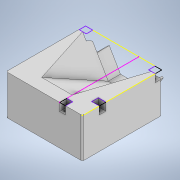
# Autodesk Inventor part: pipet tip trough
Saved by Autodesk Inventor 2020 (Build 240168000, 168)
## iProperties
Created: 2021-10-10
Part Number: pipet tip trough
Material: Generic
Document SubType Name: Modeling
Designer: pab2
Density: 1 g/cm^3
Appearance: Default
Author: pab2
Autodesk Inventor part; units mm, degrees
ref_plane "YZ Plane" through (0, 0, 0) normal (1, 0, 0) x (0, 1, 0)
ref_plane "XZ Plane" through (0, 0, 0) normal (0, 1, 0) x (-1, 0, 0)
ref_plane "XY Plane" through (0, 0, 0) normal (0, 0, 1) x (1, 0, 0)
sketch "Sketch1" plane through (0, 0, 0) normal (0, 1, 0) x (-1, 0, 0)
  line L0 (3.175, 0) -> (155.575, 0)
  line L1 (158.75, -3.175) -> (158.75, -161.925)
  line L2 (155.575, -165.1) -> (3.175, -165.1)
  line L3 (0, -161.925) -> (0, -3.175)
  arc A0 (158.75, -3.175) -> (155.575, 0) centre (155.575, -3.175) ccw
  arc A1 (155.575, -165.1) -> (158.75, -161.925) centre (155.575, -161.925) ccw
  arc A2 (0, -161.925) -> (3.175, -165.1) centre (3.175, -161.925) ccw
  arc A3 (3.175, 0) -> (0, -3.175) centre (3.175, -3.175) ccw
  point P0 (0, 0)
  point P1 (158.75, -165.1)
  point P2 (158.75, 0)
  point P3 (0, -165.1)
  dimension "d0" = 158.75
  dimension "d1" = 165.1
  dimension "d2" = 3.175
  dimension "d3" = 3.175
  dimension "d4" = 3.175
  dimension "d5" = 3.175
  constraints: 8 end point, 8 point on circle, 8 point on line, 8 tangent, 4 centre point, 2 parallel, 1 horizontal, 1 perpendicular
  measures "d0" distance of point (158.75, -165.1) point (0, -165.1)
  measures "d1" distance of point (158.75, 0) point (158.75, -165.1)
  measures "d2" radius of A0
  measures "d3" radius of A1
  measures "d4" radius of A2
  measures "d5" radius of A3
extrude "Extrusion1" add sketch "Sketch1" along normal blind 82.55
sketch "Sketch2" plane through (0, 0, 0) normal (0, -1, 0) x (1, 0, 0)
  line L0 (-3.175, -165.1) -> (-155.575, -165.1) projected
  line L1 (-6.5142, -165.1) -> (0, -165.1)
  line L2 (0, -158.9917) -> (0, -165.1)
  line L3 (0, -165.1) -> (-7.9375, -165.1)
  line L4 (-7.9375, -165.1) -> (-7.9375, -157.1625)
  line L5 (-7.9375, -157.1625) -> (0, -157.1625)
  line L6 (0, -157.1625) -> (0, -165.1)
  line L7 (-7.9375, -157.1625) -> (-149.225, -157.1625)
  line L8 (-7.9375, -157.1625) -> (-7.9375, -41.275)
  line L9 (-7.9375, -41.275) -> (-42.5857, -6.6268)
  line L10 (-7.9375, -41.275) -> (41.0625, -41.275) construction
  point P0 (0, 0)
  dimension "d8" = 7.9375
  dimension "d9" = 7.9375
  dimension "d10" = 141.2875
  dimension "d11" = 115.8875
  dimension "d12" = 49
  dimension "d13" = 135
  constraints: 20 end point, 3 horizontal, 2 parallel, 2 vertical, 1 collinear, 1 equal length, 1 perpendicular, 1 point on line
  measures "d8" distance of L4.end L5.end
  measures "d9" distance of L3.end L4.end
  measures "d10" distance of L4.end L7.end
  measures "d11" distance of L4.end L8.end
  measures "d12" distance of L8.end L9.end
  measures "d13" angle of L10 L9
hole "Hole1" at (-42.5857, 0, -6.6268) at (-7.9375, 0, -41.275) at (-7.9375, 0, -157.1625) at (-149.225, 0, -157.1625) direction (0, 1, 0) diameter 4.7625 end through all
sketch "Sketch7" plane through (-3.175, 0, -165.1) normal (0, 0, -1) x (-1, 0, 0)
  line L0 (0, 0) -> (0, 82.55) projected
  line L1 (0, 82.55) -> (44.45, 82.55)
  line L2 (152.4, 82.55) -> (0, 82.55) projected
  line L3 (0, 82.55) -> (44.45, 82.55) construction
  line L4 (44.45, 82.55) -> (107.95, 82.55)
  line L5 (107.95, 82.55) -> (107.95, 6.35)
  line L6 (107.95, 6.35) -> (44.45, 6.35)
  line L7 (44.45, 6.35) -> (44.45, 82.55)
  line L8 (44.45, 6.35) -> (0, 82.55)
  line L9 (107.95, 6.35) -> (152.4, 82.55)
  line L10 (107.95, 82.55) -> (152.4, 82.55)
  point P0 (-3.175, 0)
  dimension "d22" = 44.45
  dimension "d23" = 0
  dimension "d24" = 63.5
  dimension "d25" = 76.2
  constraints: 18 end point, 3 collinear, 2 horizontal, 2 parallel, 1 perpendicular
  measures "d22" distance of L0.end L1.end
  measures "d23" distance between parallel lines of L1 L3
  measures "d24" distance of L5.end L6.end
  measures "d25" distance of L4.end L5.end
sketch "Sketch8" plane through (0, 0, -3.175) normal (1, 0, 0) x (0, 0, -1)
  line L0 (0, 82.55) -> (-3.175, 82.55) projected
  line L1 (0, 82.55) -> (158.75, 82.55) projected
  line L2 (23.1966, 82.55) -> (161.925, 6.35)
  line L3 (161.925, 0) -> (161.925, 82.55) projected
  point P0 (-3.175, 0)
  constraints: 2 end point, 2 point on line
sweep "Sweep1" cut profiles "Sketch7" path "Sketch8" path curves L2
sketch "Sketch9" plane through (0, 82.55, 0) normal (0, 1, 0) x (1, 0, 0)
  line L0 (-3.175, 165.1) -> (-155.575, 165.1) projected
  line L1 (0, 3.175) -> (0, 161.925) projected
  line L2 (-13.8845, 165.1) -> (0, 165.1)
  line L3 (0, 165.1) -> (0, 151.6388)
  line L4 (0, 151.6388) -> (-13.8845, 151.6388)
  line L5 (-13.8845, 151.6388) -> (-13.8845, 165.1)
  line L6 (-143.876, 151.6388) -> (-158.75, 151.6388)
  line L7 (-158.75, 151.6388) -> (-158.75, 165.1)
  line L8 (-158.75, 165.1) -> (-143.876, 165.1)
  line L9 (-143.876, 165.1) -> (-143.876, 151.6388)
  line L10 (0, 3.175) -> (0, 161.925) projected
  line L11 (-15.8979, 48.8027) -> (0, 48.8027)
  line L12 (0, 48.8027) -> (0, 34.9422)
  line L13 (0, 34.9422) -> (-15.8979, 34.9422)
  line L14 (-15.8979, 34.9422) -> (-15.8979, 48.8027)
  line L15 (-47.625, 0) -> (-47.625, 165.1) projected
  line L16 (-35.1821, 14.6536) -> (-47.625, 14.6536)
  line L17 (-47.625, 14.6536) -> (-47.625, 0)
  line L18 (-47.625, 0) -> (-35.1821, 0)
  line L19 (-35.1821, 0) -> (-35.1821, 14.6536)
  point P0 (0, 0)
  point P1 (0, 48.8027)
  constraints: 32 end point, 8 parallel, 4 horizontal, 4 perpendicular, 3 point on line
extrude "Extrusion2" cut sketch "Sketch9" against normal blind 16.51 contours L2 L3 L1 L4 L5 L0 | L1 L13 L14 L11 | L16 L19 L18 L15
extrude "Extrusion3" cut sketch "Sketch9" against normal blind 80.01 contours L9 L6 L7 L8 L0
sketch "Sketch11" plane through (-3.175, 0, -165.1) normal (0, 0, -1) x (-1, 0, 0)
  line L0 (44.45, 82.55) -> (44.45, 6.35) projected
  line L1 (107.95, 6.35) -> (44.45, 6.35) projected
  line L2 (44.45, 6.35) -> (107.95, 6.35)
  line L3 (107.95, 6.35) -> (107.95, 3.175)
  line L4 (107.95, 3.175) -> (44.45, 3.175)
  line L5 (44.45, 3.175) -> (44.45, 6.35)
  line L6 (44.45, 6.35) -> (9.6308, 66.04) projected
  line L7 (21.1649, 46.2673) -> (46.3021, 3.175)
  line L8 (46.3021, 3.175) -> (43.5596, 1.5752)
  line L9 (43.5596, 1.5752) -> (18.4224, 44.6675)
  line L10 (18.4224, 44.6675) -> (21.1649, 46.2673)
  line L11 (140.701, 62.4945) -> (107.95, 6.35) projected
  line L12 (131.2351, 46.2673) -> (106.0979, 3.175)
  line L13 (106.0979, 3.175) -> (108.8404, 1.5752)
  line L14 (108.8404, 1.5752) -> (133.9776, 44.6675)
  line L15 (133.9776, 44.6675) -> (131.2351, 46.2673)
  point P0 (-3.175, 0)
  dimension "d40" = 3.175
  dimension "d41" = 3.175
  dimension "d42" = 3.175
  constraints: 24 end point, 6 parallel, 4 point on line, 3 perpendicular, 2 collinear, 1 horizontal
  measures "d40" distance of L1.start L3.end
  measures "d41" distance of L7.end L8.end
  measures "d42" distance of L13.end L12.end
extrude "Extrusion5" add sketch "Sketch11" along normal blind 25.4
body "Solid1"
